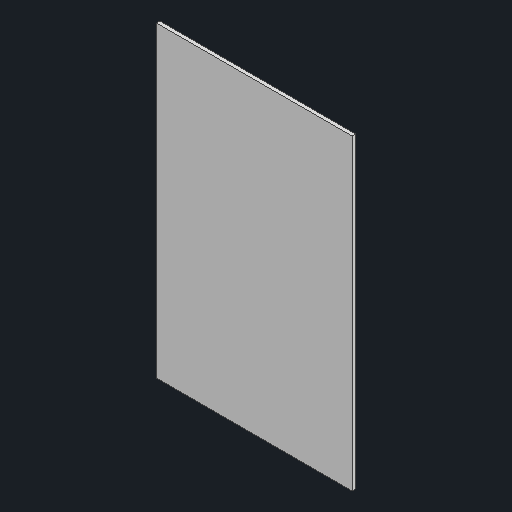
# Autodesk Inventor part: Suporte Painel1
Saved by Autodesk Inventor 2026.2 (Build 302298010, 298A)
## iProperties
Created: 2025-11-02
Part Number: Suporte Painel1
Material: Generic
Document SubType Name: Modeling
Designer: gusta
Density: 1 g/cm^3
Appearance: Default
Author: gusta
Autodesk Inventor part; units mm, degrees
ref_plane "YZ Plane" through (0, 0, 0) normal (1, 0, 0) x (0, 1, 0)
ref_plane "XZ Plane" through (0, 0, 0) normal (0, 1, 0) x (-1, 0, 0)
ref_plane "XY Plane" through (0, 0, 0) normal (0, 0, 1) x (1, 0, 0)
sketch "Sketch1" plane through (0, 0, 0) normal (0, 0, 1) x (1, 0, 0)
  line L0 (0, 0) -> (280, 0)
  line L1 (280, 0) -> (280, 440)
  line L2 (280, 440) -> (0, 440)
  line L3 (0, 440) -> (0, 0)
  dimension "d0" = 280
  dimension "d1" = 440
  constraints: 8 end point, 2 parallel, 1 horizontal, 1 perpendicular
  measures "d0" distance of L2.end L1.end
  measures "d1" distance of L1.end L0.end
extrude "Extrusion1" add sketch "Sketch1" along normal blind 5
body "Solid1"
